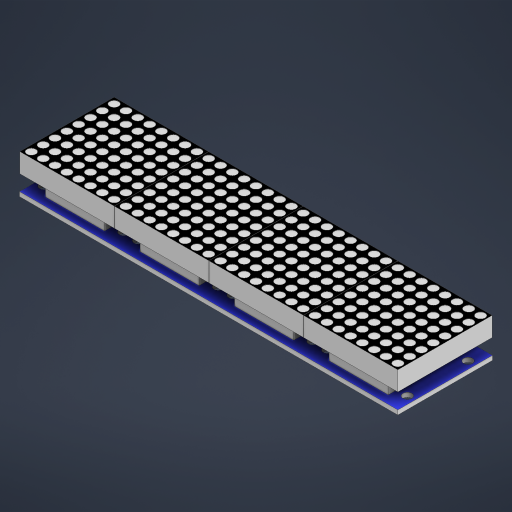
# Autodesk Inventor part: dot matrix 4
Saved by Autodesk Inventor 2024 (Build 280153000, 153)
## iProperties
Created: 2023-07-16
Part Number: dot matrix 4
Material: 일반
Document SubType Name: Modeling
Designer: 6gioc
Density: 1 g/cm^3
Appearance: 기본값
Author: 6gioc
Autodesk Inventor part; units mm, degrees
ref_plane "YZ Plane" through (0, 0, 0) normal (1, 0, 0) x (0, 1, 0)
ref_plane "XZ Plane" through (0, 0, 0) normal (0, 1, 0) x (-1, 0, 0)
ref_plane "XY Plane" through (0, 0, 0) normal (0, 0, 1) x (1, 0, 0)
sketch "스케치1" plane through (0, 0, 0) normal (0, 1, 0) x (-1, 0, 0)
  line L0 (0, 0) -> (-128, 0)
  line L1 (-128, 0) -> (-128, -32)
  line L2 (-128, -32) -> (0, -32)
  line L3 (0, -32) -> (0, 0)
  line L4 (0, -32) -> (-32, -32)
  line L5 (-32, -32) -> (-32, 0)
  line L6 (-32, 0) -> (0, 0)
  line L7 (0, 0) -> (0, -32)
  line L8 (-32, -32) -> (-64, -32)
  line L9 (-64, -32) -> (-64, 0)
  line L10 (-64, 0) -> (-32, 0)
  line L11 (-32, 0) -> (-32, -32)
  line L12 (-64, -32) -> (-96, -32)
  line L13 (-96, -32) -> (-96, 0)
  line L14 (-96, 0) -> (-64, 0)
  line L15 (-64, 0) -> (-64, -32)
  line L16 (-96, -32) -> (-128, -32)
  line L17 (-128, -32) -> (-128, 0)
  line L18 (-128, 0) -> (-96, 0)
  line L19 (-96, 0) -> (-96, -32)
  circle A0 centre (-2.5, -26.25) radius 1.5
  circle A1 centre (-2.5, -5.75) radius 1.5
  circle A2 centre (-29.5, -26.25) radius 1.5
  circle A3 centre (-29.5, -5.75) radius 1.5
  circle A4 centre (-61.5, -26.25) radius 1.5
  circle A5 centre (-61.5, -5.75) radius 1.5
  circle A6 centre (-34.5, -26.25) radius 1.5
  circle A7 centre (-34.5, -5.75) radius 1.5
  circle A8 centre (-125.5, -26.25) radius 1.5
  circle A9 centre (-125.5, -5.75) radius 1.5
  circle A10 centre (-98.5, -26.25) radius 1.5
  circle A11 centre (-98.5, -5.75) radius 1.5
  circle A12 centre (-66.5, -26.25) radius 1.5
  circle A13 centre (-93.5, -26.25) radius 1.5
  circle A14 centre (-93.5, -5.75) radius 1.5
  circle A15 centre (-66.5, -5.75) radius 1.5
  dimension "d0" = 128
  dimension "d1" = 32
  dimension "d2" = 32
  dimension "d3" = 32
  dimension "d4" = 32
  dimension "d5" = 32
  dimension "d6" = 32
  dimension "d7" = 32
  dimension "d8" = 32
  dimension "d9" = 32
  dimension "d10" = 3
  dimension "d11" = 3
  dimension "d12" = 3
  dimension "d13" = 3
  dimension "d14" = 27
  dimension "d15" = 20.5
  dimension "d16" = 2.5
  dimension "d17" = 5.75
  constraints: 40 end point, 16 centre point, 12 symmetric about line, 10 parallel, 5 horizontal, 5 perpendicular, 2 horizontal alignment, 2 vertical alignment, 12 other
  measures "d0" distance of L2.end L1.end
  measures "d1" distance of L1.end L0.end
  measures "d2" distance of L5.end L6.end
  measures "d3" distance of L4.end L5.end
  measures "d4" distance of L9.end L10.end
  measures "d5" distance of L8.end L9.end
  measures "d6" distance of L13.end L14.end
  measures "d7" distance of L12.end L13.end
  measures "d8" distance of L0.end L18.end
  measures "d9" distance of L16.end L0.end
  measures "d10" diameter of A0
  measures "d11" diameter of A1
  measures "d12" diameter of A2
  measures "d13" diameter of A3
  measures "d14" distance of A2.centre A0.centre
  measures "d15" distance of A3.centre A2.centre
  measures "d16" distance from line of L5 A2.centre
  measures "d17" distance from line of L0 A3.centre
extrude "돌출1" add sketch "스케치1" along normal blind 1.5
sketch "스케치2" plane through (0, 1.5, 0) normal (0, 1, 0) x (1, 0, 0)
  line L0 (0, 32) -> (0, 0) projected
  line L1 (0, 0) -> (128, 0) projected
  line L2 (128, 0) -> (128, 32) projected
  line L3 (128, 32) -> (0, 32) projected
  circle A0 centre (61.5, 26.25) radius 1.5 projected
  circle A1 centre (34.5, 26.25) radius 1.5 projected
  circle A2 centre (34.5, 5.75) radius 1.5 projected
  circle A3 centre (61.5, 5.75) radius 1.5 projected
  circle A4 centre (125.5, 26.25) radius 1.5 projected
  circle A5 centre (98.5, 26.25) radius 1.5 projected
  circle A6 centre (98.5, 5.75) radius 1.5 projected
  circle A7 centre (125.5, 5.75) radius 1.5 projected
  circle A8 centre (93.5, 5.75) radius 1.5 projected
  circle A9 centre (66.5, 5.75) radius 1.5 projected
  circle A10 centre (66.5, 26.25) radius 1.5 projected
  circle A11 centre (93.5, 26.25) radius 1.5 projected
  circle A12 centre (29.5, 5.75) radius 1.5 projected
  circle A13 centre (29.5, 26.25) radius 1.5 projected
  circle A14 centre (2.5, 5.75) radius 1.5 projected
  circle A15 centre (2.5, 26.25) radius 1.5 projected
  line L4 (32, 0) -> (32, 32) projected
  line L5 (64, 0) -> (64, 32) projected
  line L6 (96, 32) -> (96, 0) projected
  circle A16 centre (125.5, 5.75) radius 1.5 projected
  circle A17 centre (98.5, 5.75) radius 1.5 projected
  line L7 (0, 32) -> (0, 0) projected
  line L8 (128, 32) -> (0, 32) projected
  line L9 (128, 0) -> (128, 32) projected
  line L10 (0, 0) -> (128, 0) projected
  circle A18 centre (61.5, 26.25) radius 1.5 projected
  circle A19 centre (34.5, 26.25) radius 1.5 projected
  circle A20 centre (34.5, 5.75) radius 1.5 projected
  circle A21 centre (61.5, 5.75) radius 1.5 projected
  circle A22 centre (125.5, 26.25) radius 1.5 projected
  circle A23 centre (98.5, 26.25) radius 1.5 projected
  circle A24 centre (98.5, 5.75) radius 1.5 projected
  circle A25 centre (125.5, 5.75) radius 1.5 projected
  circle A26 centre (93.5, 5.75) radius 1.5 projected
  circle A27 centre (66.5, 5.75) radius 1.5 projected
  circle A28 centre (66.5, 26.25) radius 1.5 projected
  circle A29 centre (93.5, 26.25) radius 1.5 projected
  circle A30 centre (29.5, 5.75) radius 1.5 projected
  circle A31 centre (29.5, 26.25) radius 1.5 projected
  circle A32 centre (2.5, 5.75) radius 1.5 projected
  circle A33 centre (2.5, 26.25) radius 1.5 projected
  line L11 (6, 2.75) -> (26, 2.75)
  line L12 (26, 2.75) -> (26, 5.25)
  line L13 (26, 5.25) -> (6, 5.25)
  line L14 (6, 5.25) -> (6, 2.75)
  line L15 (6, 29.25) -> (26, 29.25)
  line L16 (26, 29.25) -> (26, 26.75)
  line L17 (26, 26.75) -> (6, 26.75)
  line L18 (6, 26.75) -> (6, 29.25)
  line L19 (58, 2.75) -> (38, 2.75)
  line L20 (38, 2.75) -> (38, 5.25)
  line L21 (38, 5.25) -> (58, 5.25)
  line L22 (58, 5.25) -> (58, 2.75)
  line L23 (58, 29.25) -> (38, 29.25)
  line L24 (38, 29.25) -> (38, 26.75)
  line L25 (38, 26.75) -> (58, 26.75)
  line L26 (58, 26.75) -> (58, 29.25)
  line L27 (122, 2.75) -> (102, 2.75)
  line L28 (102, 2.75) -> (102, 5.25)
  line L29 (102, 5.25) -> (122, 5.25)
  line L30 (122, 5.25) -> (122, 2.75)
  line L31 (122, 29.25) -> (102, 29.25)
  line L32 (102, 29.25) -> (102, 26.75)
  line L33 (102, 26.75) -> (122, 26.75)
  line L34 (122, 26.75) -> (122, 29.25)
  line L35 (90, 29.25) -> (90, 26.75)
  line L36 (70, 29.25) -> (90, 29.25)
  line L37 (70, 26.75) -> (70, 29.25)
  line L38 (90, 26.75) -> (70, 26.75)
  line L39 (90, 2.75) -> (90, 5.25)
  line L40 (90, 5.25) -> (70, 5.25)
  line L41 (70, 2.75) -> (90, 2.75)
  line L42 (70, 5.25) -> (70, 2.75)
  point P0 (6, 28)
  point P1 (6, 4)
  point P2 (58, 28)
  point P3 (58, 4)
  point P4 (122, 28)
  point P5 (122, 4)
  point P6 (70, 28)
  point P7 (70, 4)
  dimension "d20" = 20
  dimension "d21" = 2.5
  dimension "d22" = 20
  dimension "d23" = 2.5
  dimension "d24" = 21.5
  dimension "d25" = 6
  dimension "d26" = 2.75
  dimension "d27" = 2.75
  constraints: 64 end point, 30 symmetric about line, 4 parallel, 2 horizontal, 2 midpoint, 2 perpendicular, 1 vertical alignment
  measures "d20" distance of L13.end L12.end
  measures "d21" distance of L12.end L11.end
  measures "d22" distance of L16.end L17.end
  measures "d23" distance of L15.end L16.end
  measures "d24" distance between parallel lines of L13 L17
  measures "d25" horizontal distance of point (0, 0) L11.start
  measures "d26" distance between parallel lines of L1 L11
  measures "d27" distance between parallel lines of L3 L15
extrude "돌출2" add sketch "스케치2" along normal blind 5.2 contours L14 L13 L12 L11 | L15 L16 L17 L18 | L19 L20 L21 L22 | L26 L25 L24 L23 | L27 L28 L29 L30 | L34 L33 L32 L31 | L35 L38 L37 L36 | L41 L42 L40 L39
sketch "스케치3" plane through (0, 6.7, 0) normal (0, 1, 0) x (1, 0, 0)
  line L0 (0, 32) -> (0, 0) projected
  line L1 (128, 32) -> (0, 32) projected
  line L2 (128, 0) -> (128, 32) projected
  line L3 (0, 0) -> (128, 0) projected
  circle A0 centre (61.5, 26.25) radius 1.5 projected
  circle A1 centre (34.5, 26.25) radius 1.5 projected
  circle A2 centre (34.5, 5.75) radius 1.5 projected
  circle A3 centre (61.5, 5.75) radius 1.5 projected
  circle A4 centre (125.5, 26.25) radius 1.5 projected
  circle A5 centre (98.5, 26.25) radius 1.5 projected
  circle A6 centre (98.5, 5.75) radius 1.5 projected
  circle A7 centre (125.5, 5.75) radius 1.5 projected
  circle A8 centre (93.5, 5.75) radius 1.5 projected
  circle A9 centre (66.5, 5.75) radius 1.5 projected
  circle A10 centre (66.5, 26.25) radius 1.5 projected
  circle A11 centre (93.5, 26.25) radius 1.5 projected
  circle A12 centre (29.5, 5.75) radius 1.5 projected
  circle A13 centre (29.5, 26.25) radius 1.5 projected
  circle A14 centre (2.5, 5.75) radius 1.5 projected
  circle A15 centre (2.5, 26.25) radius 1.5 projected
  line L4 (32, 0) -> (32, 32) projected
  line L5 (64, 32) -> (64, 0) projected
  line L6 (96, 32) -> (96, 0) projected
  line L7 (0.05, 31.95) -> (31.95, 31.95)
  line L8 (31.95, 31.95) -> (31.95, 0.05)
  line L9 (31.95, 0.05) -> (0.05, 0.05)
  line L10 (0.05, 0.05) -> (0.05, 31.95)
  line L11 (63.95, 31.95) -> (32.05, 31.95)
  line L12 (32.05, 31.95) -> (32.05, 0.05)
  line L13 (32.05, 0.05) -> (63.95, 0.05)
  line L14 (63.95, 0.05) -> (63.95, 31.95)
  line L15 (127.95, 31.95) -> (96.05, 31.95)
  line L16 (96.05, 31.95) -> (96.05, 0.05)
  line L17 (96.05, 0.05) -> (127.95, 0.05)
  line L18 (127.95, 0.05) -> (127.95, 31.95)
  line L19 (64.05, 31.95) -> (95.95, 31.95)
  line L20 (95.95, 31.95) -> (95.95, 0.05)
  line L21 (95.95, 0.05) -> (64.05, 0.05)
  line L22 (64.05, 0.05) -> (64.05, 31.95)
  dimension "d30" = 31.9
  dimension "d31" = 31.9
  dimension "d32" = 0.05
  dimension "d33" = 0.05
  constraints: 32 end point, 12 symmetric about line, 2 parallel, 1 horizontal, 1 perpendicular
  measures "d30" distance of L8.end L9.end
  measures "d31" distance of L7.end L8.end
  measures "d32" distance between parallel lines of L0 L10
  measures "d33" distance between parallel lines of L1 L7
extrude "돌출3" add sketch "스케치3" along normal blind 6.5 contours A0 | A1 | A2 | A3 | A4 | A5 | A6 | A7 | A8 | A9 | A10 | A11 | A12 | A13 | A14 | A15 | L7 L8 L9 L10 | L14 L13 L12 L11 | L18 L17 L16 L15 | L19 L20 L21 L22
sketch "스케치4" plane through (0, 13.2, 0) normal (0, 1, 0) x (1, 0, 0)
  line L0 (0.05, 0.05) -> (31.95, 0.05) projected
  line L1 (31.95, 0.05) -> (31.95, 31.95) projected
  line L2 (31.95, 31.95) -> (0.05, 31.95) projected
  line L3 (0.05, 31.95) -> (0.05, 0.05) projected
  circle A0 centre (2, 30) radius 1.5
  circle A1 centre (6, 30) radius 1.5
  circle A2 centre (10, 30) radius 1.5
  circle A3 centre (14, 30) radius 1.5
  circle A4 centre (18, 30) radius 1.5
  circle A5 centre (22, 30) radius 1.5
  circle A6 centre (26, 30) radius 1.5
  circle A7 centre (30, 30) radius 1.5
  circle A8 centre (2, 26) radius 1.5
  circle A9 centre (6, 26) radius 1.5
  circle A10 centre (10, 26) radius 1.5
  circle A11 centre (14, 26) radius 1.5
  circle A12 centre (18, 26) radius 1.5
  circle A13 centre (22, 26) radius 1.5
  circle A14 centre (26, 26) radius 1.5
  circle A15 centre (30, 26) radius 1.5
  line L4 (31.95, 47.95) -> (31.95, 16.05)
  circle A16 centre (6, 22) radius 1.5
  circle A17 centre (2, 22) radius 1.5
  circle A18 centre (10, 22) radius 1.5
  circle A19 centre (18, 22) radius 1.5
  circle A20 centre (22, 22) radius 1.5
  circle A21 centre (26, 22) radius 1.5
  circle A22 centre (30, 22) radius 1.5
  circle A23 centre (14, 22) radius 1.5
  circle A24 centre (6, 14) radius 1.5
  circle A25 centre (2, 14) radius 1.5
  circle A26 centre (10, 14) radius 1.5
  circle A27 centre (18, 14) radius 1.5
  circle A28 centre (22, 14) radius 1.5
  circle A29 centre (26, 14) radius 1.5
  circle A30 centre (30, 14) radius 1.5
  circle A31 centre (14, 14) radius 1.5
  circle A32 centre (18, 18) radius 1.5
  circle A33 centre (14, 18) radius 1.5
  circle A34 centre (30, 18) radius 1.5
  circle A35 centre (22, 18) radius 1.5
  circle A36 centre (26, 18) radius 1.5
  circle A37 centre (2, 18) radius 1.5
  circle A38 centre (10, 18) radius 1.5
  circle A39 centre (6, 18) radius 1.5
  line L5 (0.05, 0) -> (31.95, 0)
  circle A40 centre (18, 2) radius 1.5
  circle A41 centre (14, 2) radius 1.5
  circle A42 centre (30, 2) radius 1.5
  circle A43 centre (22, 2) radius 1.5
  circle A44 centre (26, 2) radius 1.5
  circle A45 centre (2, 2) radius 1.5
  circle A46 centre (10, 2) radius 1.5
  circle A47 centre (6, 2) radius 1.5
  circle A48 centre (2, 6) radius 1.5
  circle A49 centre (10, 6) radius 1.5
  circle A50 centre (2, 10) radius 1.5
  circle A51 centre (6, 6) radius 1.5
  circle A52 centre (10, 10) radius 1.5
  circle A53 centre (6, 10) radius 1.5
  circle A54 centre (14, 10) radius 1.5
  circle A55 centre (18, 10) radius 1.5
  circle A56 centre (18, 6) radius 1.5
  circle A57 centre (14, 6) radius 1.5
  circle A58 centre (22, 6) radius 1.5
  circle A59 centre (22, 10) radius 1.5
  circle A60 centre (26, 6) radius 1.5
  circle A61 centre (26, 10) radius 1.5
  circle A62 centre (30, 10) radius 1.5
  circle A63 centre (30, 6) radius 1.5
  line L6 (32, 0) -> (32, 32) projected
  line L7 (64, 0) -> (64, 32) projected
  line L8 (96, 32) -> (96, 0) projected
  circle A64 centre (62, 30) radius 1.5
  circle A65 centre (58, 30) radius 1.5
  circle A66 centre (54, 30) radius 1.5
  circle A67 centre (50, 30) radius 1.5
  circle A68 centre (46, 30) radius 1.5
  circle A69 centre (42, 30) radius 1.5
  circle A70 centre (38, 30) radius 1.5
  circle A71 centre (34, 30) radius 1.5
  circle A72 centre (58, 26) radius 1.5
  circle A73 centre (62, 26) radius 1.5
  circle A74 centre (54, 26) radius 1.5
  circle A75 centre (46, 26) radius 1.5
  circle A76 centre (42, 26) radius 1.5
  circle A77 centre (38, 26) radius 1.5
  circle A78 centre (34, 26) radius 1.5
  circle A79 centre (50, 26) radius 1.5
  circle A80 centre (46, 22) radius 1.5
  circle A81 centre (50, 22) radius 1.5
  circle A82 centre (34, 22) radius 1.5
  circle A83 centre (42, 22) radius 1.5
  circle A84 centre (38, 22) radius 1.5
  circle A85 centre (62, 22) radius 1.5
  circle A86 centre (54, 22) radius 1.5
  circle A87 centre (58, 22) radius 1.5
  circle A88 centre (62, 18) radius 1.5
  circle A89 centre (54, 18) radius 1.5
  circle A90 centre (62, 14) radius 1.5
  circle A91 centre (58, 18) radius 1.5
  circle A92 centre (54, 14) radius 1.5
  circle A93 centre (58, 14) radius 1.5
  circle A94 centre (50, 14) radius 1.5
  circle A95 centre (46, 14) radius 1.5
  circle A96 centre (46, 18) radius 1.5
  circle A97 centre (50, 18) radius 1.5
  circle A98 centre (42, 18) radius 1.5
  circle A99 centre (42, 14) radius 1.5
  circle A100 centre (38, 18) radius 1.5
  circle A101 centre (38, 14) radius 1.5
  circle A102 centre (34, 14) radius 1.5
  circle A103 centre (34, 18) radius 1.5
  circle A104 centre (42, 2) radius 1.5
  circle A105 centre (42, 10) radius 1.5
  circle A106 centre (42, 6) radius 1.5
  circle A107 centre (38, 6) radius 1.5
  circle A108 centre (38, 10) radius 1.5
  circle A109 centre (38, 2) radius 1.5
  circle A110 centre (34, 10) radius 1.5
  circle A111 centre (46, 2) radius 1.5
  circle A112 centre (46, 10) radius 1.5
  circle A113 centre (46, 6) radius 1.5
  circle A114 centre (50, 2) radius 1.5
  circle A115 centre (50, 6) radius 1.5
  circle A116 centre (50, 10) radius 1.5
  circle A117 centre (62, 2) radius 1.5
  circle A118 centre (54, 2) radius 1.5
  circle A119 centre (58, 2) radius 1.5
  circle A120 centre (62, 6) radius 1.5
  circle A121 centre (54, 6) radius 1.5
  circle A122 centre (54, 10) radius 1.5
  circle A123 centre (58, 6) radius 1.5
  circle A124 centre (58, 10) radius 1.5
  circle A125 centre (62, 10) radius 1.5
  circle A126 centre (34, 6) radius 1.5
  circle A127 centre (34, 2) radius 1.5
  line L9 (96.05, 0.05) -> (96.05, 31.95)
  line L10 (96.05, 31.95) -> (127.95, 31.95)
  circle A128 centre (126, 30) radius 1.5
  circle A129 centre (122, 30) radius 1.5
  circle A130 centre (118, 30) radius 1.5
  circle A131 centre (114, 30) radius 1.5
  circle A132 centre (110, 30) radius 1.5
  circle A133 centre (106, 30) radius 1.5
  circle A134 centre (102, 30) radius 1.5
  circle A135 centre (98, 30) radius 1.5
  circle A136 centre (122, 26) radius 1.5
  circle A137 centre (126, 26) radius 1.5
  circle A138 centre (118, 26) radius 1.5
  circle A139 centre (110, 26) radius 1.5
  circle A140 centre (106, 26) radius 1.5
  circle A141 centre (102, 26) radius 1.5
  circle A142 centre (98, 26) radius 1.5
  circle A143 centre (114, 26) radius 1.5
  line L11 (96.05, 47.95) -> (96.05, 16.05)
  circle A144 centre (110, 22) radius 1.5
  circle A145 centre (114, 22) radius 1.5
  circle A146 centre (98, 22) radius 1.5
  circle A147 centre (106, 22) radius 1.5
  circle A148 centre (102, 22) radius 1.5
  circle A149 centre (126, 22) radius 1.5
  circle A150 centre (118, 22) radius 1.5
  circle A151 centre (122, 22) radius 1.5
  circle A152 centre (126, 18) radius 1.5
  circle A153 centre (118, 18) radius 1.5
  circle A154 centre (126, 14) radius 1.5
  circle A155 centre (122, 18) radius 1.5
  circle A156 centre (118, 14) radius 1.5
  circle A157 centre (122, 14) radius 1.5
  circle A158 centre (114, 14) radius 1.5
  circle A159 centre (110, 14) radius 1.5
  circle A160 centre (110, 18) radius 1.5
  circle A161 centre (114, 18) radius 1.5
  circle A162 centre (106, 18) radius 1.5
  circle A163 centre (106, 14) radius 1.5
  circle A164 centre (102, 18) radius 1.5
  circle A165 centre (102, 14) radius 1.5
  circle A166 centre (98, 14) radius 1.5
  circle A167 centre (98, 18) radius 1.5
  circle A168 centre (106, 2) radius 1.5
  circle A169 centre (106, 10) radius 1.5
  circle A170 centre (106, 6) radius 1.5
  circle A171 centre (102, 6) radius 1.5
  circle A172 centre (102, 10) radius 1.5
  circle A173 centre (102, 2) radius 1.5
  circle A174 centre (98, 10) radius 1.5
  circle A175 centre (110, 2) radius 1.5
  circle A176 centre (110, 10) radius 1.5
  circle A177 centre (110, 6) radius 1.5
  circle A178 centre (114, 2) radius 1.5
  circle A179 centre (114, 6) radius 1.5
  circle A180 centre (114, 10) radius 1.5
  circle A181 centre (126, 2) radius 1.5
  circle A182 centre (118, 2) radius 1.5
  circle A183 centre (122, 2) radius 1.5
  circle A184 centre (126, 6) radius 1.5
  circle A185 centre (118, 6) radius 1.5
  circle A186 centre (118, 10) radius 1.5
  circle A187 centre (122, 6) radius 1.5
  circle A188 centre (122, 10) radius 1.5
  circle A189 centre (126, 10) radius 1.5
  circle A190 centre (98, 6) radius 1.5
  circle A191 centre (98, 2) radius 1.5
  line L12 (96, 0) -> (96, 32)
  circle A192 centre (70, 26) radius 1.5
  circle A193 centre (66, 30) radius 1.5
  circle A194 centre (74, 26) radius 1.5
  circle A195 centre (66, 26) radius 1.5
  circle A196 centre (70, 22) radius 1.5
  circle A197 centre (74, 22) radius 1.5
  circle A198 centre (66, 22) radius 1.5
  circle A199 centre (70, 18) radius 1.5
  circle A200 centre (74, 18) radius 1.5
  circle A201 centre (66, 18) radius 1.5
  circle A202 centre (74, 14) radius 1.5
  circle A203 centre (70, 14) radius 1.5
  circle A204 centre (66, 14) radius 1.5
  circle A205 centre (86, 26) radius 1.5
  circle A206 centre (86, 22) radius 1.5
  circle A207 centre (90, 18) radius 1.5
  circle A208 centre (82, 26) radius 1.5
  circle A209 centre (82, 22) radius 1.5
  circle A210 centre (78, 26) radius 1.5
  circle A211 centre (90, 14) radius 1.5
  circle A212 centre (78, 22) radius 1.5
  circle A213 centre (86, 18) radius 1.5
  circle A214 centre (86, 14) radius 1.5
  circle A215 centre (82, 18) radius 1.5
  circle A216 centre (78, 18) radius 1.5
  circle A217 centre (82, 14) radius 1.5
  circle A218 centre (78, 14) radius 1.5
  circle A219 centre (86, 10) radius 1.5
  circle A220 centre (90, 10) radius 1.5
  circle A221 centre (86, 6) radius 1.5
  circle A222 centre (90, 6) radius 1.5
  circle A223 centre (90, 2) radius 1.5
  circle A224 centre (86, 2) radius 1.5
  circle A225 centre (70, 30) radius 1.5
  circle A226 centre (74, 30) radius 1.5
  circle A227 centre (78, 30) radius 1.5
  circle A228 centre (82, 30) radius 1.5
  circle A229 centre (86, 30) radius 1.5
  circle A230 centre (90, 26) radius 1.5
  circle A231 centre (90, 30) radius 1.5
  circle A232 centre (90, 22) radius 1.5
  circle A233 centre (82, 10) radius 1.5
  circle A234 centre (82, 6) radius 1.5
  circle A235 centre (78, 10) radius 1.5
  circle A236 centre (78, 6) radius 1.5
  circle A237 centre (78, 2) radius 1.5
  circle A238 centre (82, 2) radius 1.5
  circle A239 centre (70, 10) radius 1.5
  circle A240 centre (66, 10) radius 1.5
  circle A241 centre (74, 10) radius 1.5
  circle A242 centre (70, 6) radius 1.5
  circle A243 centre (74, 6) radius 1.5
  circle A244 centre (66, 6) radius 1.5
  circle A245 centre (74, 2) radius 1.5
  circle A246 centre (70, 2) radius 1.5
  circle A247 centre (66, 2) radius 1.5
  circle A248 centre (94, 30) radius 1.5
  circle A249 centre (94, 26) radius 1.5
  circle A250 centre (94, 22) radius 1.5
  circle A251 centre (94, 14) radius 1.5
  circle A252 centre (94, 18) radius 1.5
  circle A253 centre (94, 10) radius 1.5
  circle A254 centre (94, 6) radius 1.5
  circle A255 centre (94, 2) radius 1.5
  point P0 (0, 0)
  dimension "d36" = 31.9
  dimension "d37" = 3
  dimension "d38" = 3
  dimension "d39" = 3
  dimension "d40" = 3
  dimension "d41" = 3
  dimension "d42" = 3
  dimension "d43" = 3
  dimension "d44" = 3
  dimension "d45" = 4
  dimension "d46" = 4
  dimension "d47" = 4
  dimension "d48" = 4
  dimension "d49" = 4
  dimension "d50" = 4
  dimension "d51" = 4
  dimension "d52" = 28
  dimension "d53" = 1.95
  dimension "d54" = 1.95
  constraints: 256 centre point, 197 symmetric about line, 12 end point, 7 horizontal alignment, 192 other
  measures "d36" distance of L1.end L2.end
  measures "d37" diameter of A0
  measures "d38" diameter of A1
  measures "d39" diameter of A2
  measures "d40" diameter of A3
  measures "d41" diameter of A4
  measures "d42" diameter of A5
  measures "d43" diameter of A6
  measures "d44" diameter of A7
  measures "d45" distance of A1.centre A0.centre
  measures "d46" distance of A2.centre A1.centre
  measures "d47" distance of A3.centre A2.centre
  measures "d48" distance of A4.centre A3.centre
  measures "d49" distance of A5.centre A4.centre
  measures "d50" distance of A6.centre A5.centre
  measures "d51" distance of A7.centre A6.centre
  measures "d52" distance between centres of A7 A0
  measures "d53" distance from line of L1 A7.centre
  measures "d54" distance from line of L2 A7.centre
extrude "돌출4" cut sketch "스케치4" against normal blind 0.1 contours A0 | A1 | A2 | A3 | A4 | A5 | A6 | A7 | A8 | A9 | A10 | A11 | A12 | A13 | A14 | A15 | A16 | A17 | A18 | A19 | A20 | A21 | A22 | A23 | A24 | A25 | A26 | A27 | A28 | A29 | A30 | A31 | A32 | A33 | A34 | A35 | A36 | A37 | A38 | A39 | A40 | A41 | A42 | A43 | A44 | A45 | A46 | A47 | A48 | A49 | A50 | A51 | A52 | A53 | A54 | A55 | A56 | A57 | A58 | A59 | A60 | A61 | A62 | A63 | A64 | A65 | A66 | A67 | A68 | A69 | A70 | A71 | A72 | A73 | A74 | A75 | A76 | A77 | A78 | A79 | A80 | A81 | A82 | A83 | A84 | A85 | A86 | A87 | A88 | A89 | A90 | A91 | A92 | A93 | A94 | A95 | A96 | A97 | A98 | A99 | A100 | A101 | A102 | A103 | A104 | A105 | A106 | A107 | A108 | A109 | A110 | A111 | A112 | A113 | A114 | A115 | A116 | A117 | A118 | A119 | A120 | A121 | A122 | A123 | A124 | A125 | A126 | A127 | A128 | A129 | A130 | A131 | A132 | A133 | A134 | A135 | A136 | A137 | A138 | A139 | A140 | A141 | A142 | A143 | A144 | A145 | A146 | A147 | A148 | A149 | A150 | A151 | A152 | A153 | A154 | A155 | A156 | A157 | A158 | A159 | A160 | A161 | A162 | A163 | A164 | A165 | A166 | A167 | A168 | A169 | A170 | A171 | A172 | A173 | A174 | A175 | A176 | A177 | A178 | A179 | A180 | A181 | A182 | A183 | A184 | A185 | A186 | A187 | A188 | A189 | A190 | A191 | A192 | A193 | A194 | A195 | A196 | A197 | A198 | A199 | A200 | A201 | A202 | A203 | A204 | A205 | A206 | A207 | A208 | A209 | A210 | A211 | A212 | A213 | A214 | A215 | A216 | A217 | A218 | A219 | A220 | A221 | A222 | A223 | A224 | A225 | A226 | A227 | A228 | A229 | A230 | A231 | A232 | A233 | A234 | A235 | A236 | A237 | A238 | A239 | A240 | A241 | A242 | A243 | A244 | A245 | A246 | A247 | A248 | A249 | A250 | A251 | A252 | A253 | A254 | A255
